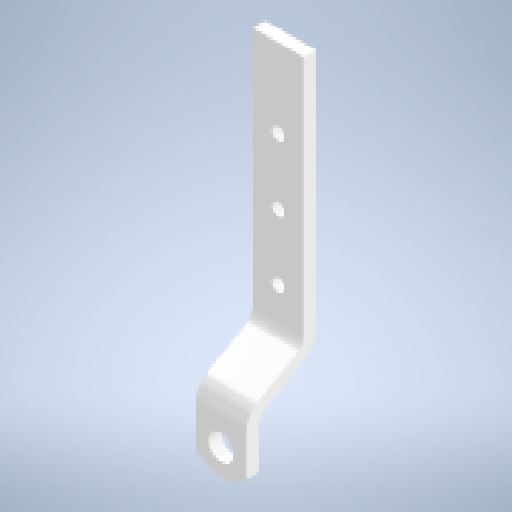
# Autodesk Inventor part: Printhead Endstop Cable Guide Plate
Saved by Autodesk Inventor 2024 (Build 280153000, 153)
## iProperties
Created: 2025-01-19
Part Number: Printhead Endstop Cable Guide Plate
Material: Aluminum 6061
Document SubType Name: Sheet Metal
Designer: Ishaan
Density: 2.7 g/cm^3
Sheet Metal Rule: SendCutSend_1-8_Alu
Appearance: Aluminum - Flat
Author: Ishaan
Autodesk Inventor part; units mm, degrees
ref_plane "YZ Plane" through (0, 0, 0) normal (1, 0, 0) x (0, 1, 0)
ref_plane "XZ Plane" through (0, 0, 0) normal (0, 1, 0) x (-1, 0, 0)
ref_plane "XY Plane" through (0, 0, 0) normal (0, 0, 1) x (1, 0, 0)
sketch "Sketch1" plane through (0, 0, 0) normal (0, 0, 1) x (1, 0, 0)
  line L0 (6.5, -25) -> (-6.5, -25)
  line L1 (-6.5, -25) -> (-6.5, 25)
  line L2 (-6.5, 25) -> (6.5, 25)
  line L3 (6.5, 25) -> (6.5, -25)
  line L4 (6.5, -25) -> (-6.5, 25) construction
  line L5 (-6.5, -25) -> (6.5, 25) construction
  line L6 (0, 16.75) -> (0, -16.75) construction
  point P0 (0, 0)
  dimension "d0" = 50
  dimension "d1" = 13
  dimension "d2" = 33.5
  constraints: 14 end point, 3 midpoint, 2 coincident, 2 parallel, 1 horizontal, 1 perpendicular, 1 vertical
  measures "d0" distance of L0.end L1.end
  measures "d1" distance of L0.start L0.end
  measures "d2" distance of L6.start L6.end
extrude "Plate1" add sketch "Sketch1" along normal blind 3.175
hole "Hole1" at (0, 0, 0) at (0, 16.75, 0) at (0, -16.75, 0) direction (0, 0, 1) diameter 3.3 end through all
sketch "Sketch2" plane through (6.5, -27.7496, 4.7625) normal (0, -0.8660254, -0.5) x (1, 0, 0)
  line L0 (-13, 0) -> (0, 0)
  line L1 (0, 0) -> (0, 11.3338)
  line L2 (0, 11.3338) -> (-13, 11.3338)
  line L3 (-13, 11.3338) -> (-13, 0)
  constraints: 6 end point, 1 horizontal, 1 perpendicular, 1 vertical
edge flange "Flange1" height 15 angle 60 thickness 3.175 bend radius 3.175 thickness toward (0, -0.8660254, -0.5) relief tear relief width 3.175 relief depth 1.5875 edges at (0, -25, 3.175) wall of the first edge with corners at (-6.5, -27.7496, 4.7625) (6.5, -27.7496, 4.7625) (6.5, -33.4165, 14.5779) (-6.5, -33.4165, 14.5779)
bend "Bend1"
corner "Corner1"
sketch "Sketch3" plane through (-6.5, -38.9158, 14.5779) normal (0, 0, 1) x (1, 0, 0)
  line L0 (13, 0) -> (0, 0)
  line L1 (0, 0) -> (0, -16.3338)
  line L2 (0, -16.3338) -> (13, -16.3338)
  line L3 (13, -16.3338) -> (13, 0)
  constraints: 6 end point, 1 horizontal, 1 perpendicular, 1 vertical
edge flange "Flange2" height 20 angle 60 thickness 3.175 bend radius 3.175 thickness toward (0, 0, 1) relief tear relief width 3.175 relief depth 1.5875 edges at (0, -36.1662, 12.9904) wall of the first edge with corners at (6.5, -38.9158, 14.5779) (-6.5, -38.9158, 14.5779) (-6.5, -55.2496, 14.5779) (6.5, -55.2496, 14.5779)
bend "Bend2"
corner "Corner2"
sketch "Sketch4" plane through (-6.5, 25, 0) normal (0, 1, 0) x (1, 0, 0)
  line L0 (0, -3.175) -> (13, -3.175) projected
  line L1 (13, 0) -> (13, -3.175) projected
  line L2 (13, 0) -> (0, 0) projected
  line L3 (0, 0) -> (0, -3.175) projected
  point P0 (6.5, 0)
extrude "Extrusion1" add sketch "Sketch4" along normal blind 12
sketch "Sketch5" plane through (-6.5, -55.2496, 17.7529) normal (0, 0, 1) x (1, 0, 0)
  circle A0 centre (6.5, 9.7496) radius 6.5
  line L0 (0, 0) -> (0, 16.3338) construction
  line L1 (0, 9.7496) -> (0, 5.4065)
  line L2 (0, 5.4065) -> (6.5, 2.7141)
  line L3 (6.5, 2.7141) -> (13, 5.4065)
  line L4 (13, 5.4065) -> (13, 9.7496)
  line L5 (13, 16.3338) -> (13, 0) construction
  line L6 (13, 16.3338) -> (0, 16.3338) projected
  line L7 (0, 0) -> (0, 16.3338) projected
  line L8 (13, 0) -> (0, 0) projected
  line L9 (13, 16.3338) -> (13, 0) projected
  point P0 (6.5, 55.2496)
  point P1 (13, 5.4065)
  point P2 (8.9874, 3.7444)
  point P3 (4.0126, 3.7444)
  point P4 (0, 5.4065)
  dimension "d33" = 45.5
  dimension "d34" = 135
  constraints: 8 end point, 5 tangent, 2 point on circle, 2 point on line, 1 centre point, 1 collinear, 1 horizontal alignment, 1 vertical alignment
  measures "d33" distance of point (6.5, 55.25) A0.centre
  measures "d34" angle of L3 L2
extrude "Extrusion2" cut sketch "Sketch5" against normal through all contours L3 L2 A0 | L3 L9 L8 L7 L2
fillet "Fillet1" radius 1 2 edges at (-6.5, -49.8432, 16.1654) (6.5, -49.8432, 16.1654)
sketch "Sketch6" plane through (-6.5, -38.9158, 17.7529) normal (0, 0, 1) x (1, 0, 0)
  arc A0 (4.0126, -12.5894) -> (8.9874, -12.5894) centre (6.5, -6.5842) ccw projected
  point P0 (6.5, 38.9158)
  constraints: 1 coincident
hole "Hole2" at (0, -45.5, 17.7529) direction (0, 0, -1) diameter 6.4 end through all
equation "\"d9\" = Thickness"
equation "\"d43\" = Thickness"
equation "\"d3\" = Thickness"
equation "\"d11\" = BendReliefWidth"
equation "\"d12\" = BendReliefDepth"
equation "\"d13\" = MinimumRemnant"
equation "\"d14\" = TransitionRadius"
equation "\"d17\" = BendRadius"
equation "\"d18\" = CornerReliefSize"
equation "\"d19\" = GapSize"
equation "\"d20\" = JacobiRadiusSize"
equation "\"d21\" = BendReliefWidth"
equation "\"d22\" = BendReliefDepth"
equation "\"d23\" = MinimumRemnant"
equation "\"d24\" = TransitionRadius"
equation "\"d27\" = BendRadius"
equation "\"d28\" = CornerReliefSize"
equation "\"d29\" = GapSize"
equation "\"d30\" = JacobiRadiusSize"
equation "\"BendReliefWidth\" = Thickness"
equation "\"BendReliefDepth\" = 0.5 * Thickness"
equation "\"CornerReliefSize\" = 4 * Thickness"
equation "\"MinimumRemnant\" = 2 * Thickness"
equation "\"TransitionRadius\" = BendRadius"
equation "\"JacobiRadiusSize\" = BendRadius"
equation "\"GapSize\" = Thickness"
equation "\"Thickness\" = 3.175"
equation "\"BendRadius\" = 3.175"
body "Solid1"
